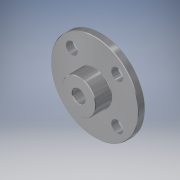
# Autodesk Inventor part: 08-0005
Saved by Autodesk Inventor 2017.1 (Build 211199000, 199)
## iProperties
Category: Wheel Service Pack
Company: Autodesk Inc.
Created: 2014-11-30
Part Number: 08-0005
Material: Aluminum 6061
Document SubType Name: Modeling
Designer: Matrix
Density: 2.7 g/cm^3
Appearance: Aluminum - Polished
Catalog Web Link: http://matrixrobotics.com/
Vendor: Matrix
Author: Autodesk Inc.
Autodesk Inventor part; units mm, degrees
ref_plane "YZ Plane" through (0, 0, 0) normal (1, 0, 0) x (0, 1, 0)
ref_plane "XZ Plane" through (0, 0, 0) normal (0, 1, 0) x (-1, 0, 0)
ref_plane "XY Plane" through (0, 0, 0) normal (0, 0, 1) x (1, 0, 0)
sketch "Sketch1" plane through (0, 0, 0) normal (0, 1, 0) x (-1, 0, 0)
  circle A0 centre (0, 0) radius 15.5
  dimension "d0" = 31
  constraints: 1 centre point, 1 coincident
  measures "d0" diameter of A0
extrude "Extrusion1" add sketch "Sketch1" against normal blind 2.4
sketch "Sketch2" plane through (0, 0, 0) normal (0, 1, 0) x (1, 0, 0)
  circle A0 centre (0, 0) radius 6
  dimension "d3" = 12
  constraints: 1 centre point, 1 coincident
  measures "d3" diameter of A0
extrude "Extrusion2" add sketch "Sketch2" along normal blind 5.6
sketch "Sketch3" plane through (0, 0, 0) normal (0, 1, 0) x (1, 0, 0)
  circle A0 centre (0, 0) radius 2.1
  circle A1 centre (7.9999, -7.9999) radius 2.1
  circle A2 centre (7.9999, 7.9999) radius 2.1
  circle A3 centre (-7.9999, 7.9999) radius 2.1
  circle A4 centre (-7.9999, -7.9999) radius 2.1
  circle A5 centre (0, 0) radius 6.1
  circle A6 centre (0, 0) radius 15.4
  point P0 (0, 0)
  constraints: 7 centre point
extrude "Extrusion3" cut sketch "Sketch3" against normal blind 5.6 contours A1 | A2 | A3 | A4
sketch "Sketch4" plane through (0, 5.6, 0) normal (0, 1, 0) x (1, 0, 0)
  point P0 (0, 0)
hole "Hole1" at (0, 5.6, 0) direction (0, -1, 0) diameter 4.5 end through all
fillet "Fillet1" radius 0.2 1 edges at (-6, 0, 0)
chamfer "Chamfer1" distance 0.2 angle 45 4 edges at (15.5, -2.4, 0) (15.5, 0, 0) (-6, 5.6, 0) (0, 5.6, -2.25)
body "Solid1"
